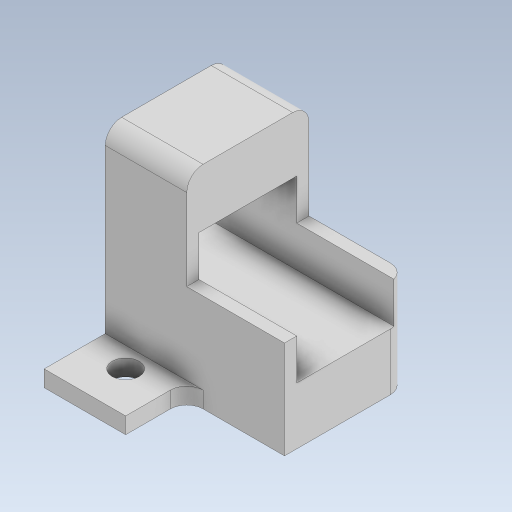
# Autodesk Inventor part: Bracket Motor Pendorong
Saved by Autodesk Inventor 2023.5 (Build 275446000, 446)
## iProperties
Created: 2025-10-12
Part Number: Bracket Motor Pendorong
Material: Generic
Document SubType Name: Modeling
Designer: Guntur
Density: 1 g/cm^3
Appearance: Default
Author: Guntur
Autodesk Inventor part; units mm, degrees
ref_plane "YZ Plane" through (0, 0, 0) normal (1, 0, 0) x (0, 1, 0)
ref_plane "XZ Plane" through (0, 0, 0) normal (0, 1, 0) x (-1, 0, 0)
ref_plane "XY Plane" through (0, 0, 0) normal (0, 0, 1) x (1, 0, 0)
sketch "Sketch1" plane through (0, 0, 0) normal (0, 1, 0) x (-1, 0, 0)
  circle A0 centre (0, -10) radius 1.65
  circle A1 centre (0, 10) radius 1.65
  line L0 (0, 0) -> (-5, 0)
  line L1 (-5, 0) -> (-5, -15)
  line L2 (-5, -15) -> (0, -15)
  line L3 (0, -15) -> (0, 0)
  line L4 (0, 0) -> (5, 0)
  line L5 (5, 0) -> (5, -15)
  line L6 (5, -15) -> (0, -15)
  line L7 (0, -15) -> (0, 0)
  line L8 (5, 0) -> (-5, 0)
  line L9 (-5, 0) -> (-5, 15)
  line L10 (-5, 15) -> (5, 15)
  line L11 (5, 15) -> (5, 0)
  line L12 (5, 7.5) -> (-5, 7.5)
  line L13 (-5, 7.5) -> (-5, -7.5)
  line L14 (-5, -7.5) -> (5, -7.5)
  line L15 (5, -7.5) -> (5, 7.5)
  line L16 (5, 7.5) -> (-5, -7.5) construction
  line L17 (-5, 7.5) -> (5, -7.5) construction
  dimension "d3" = 3.3
  dimension "d6" = 3.3
  constraints: 36 end point, 8 parallel, 4 horizontal, 4 perpendicular, 3 midpoint, 2 centre point, 1 coincident, 1 point on line
  measures "d3" diameter of A0
  measures "d6" diameter of A1
extrude "Extrusion1" add sketch "Sketch1" along normal blind 2 contours A0 L3 L14 L5 L6 | A0 L3 L2 L1 L14 | L9 L10 L11 L12
extrude "Extrusion2" add sketch "Sketch1" along normal blind 24 contours L14 L1 L0 L3 | L3 L4 L5 L14 | L0 L9 L12 L11 L4
sketch "Sketch2" plane through (5, 0, 15) normal (1, 0, 0) x (0, 0, -1)
  line L0 (9, 17) -> (21, 17)
  line L1 (21, 17) -> (21, 7)
  line L2 (21, 7) -> (9, 7)
  line L3 (9, 7) -> (9, 17)
  line L4 (9, 17) -> (21, 7) construction
  line L5 (21, 17) -> (9, 7) construction
  line L6 (7.5, 24) -> (22.5, 24) projected
  line L7 (7.5, 2) -> (7.5, 24) projected
  line L8 (30, 0) -> (0, 0) projected
  line L9 (7.5, 12) -> (22.5, 12)
  line L10 (22.5, 12) -> (22.5, 0)
  line L11 (22.5, 0) -> (7.5, 0)
  line L12 (7.5, 0) -> (7.5, 12)
  point P0 (15, 0)
  point P1 (15, 12)
  point P2 (7.5, 0)
  point P3 (21, 12)
  point P4 (9, 12)
  point P5 (9, 12)
  point P6 (21, 12)
  dimension "d13" = 7
  dimension "d14" = 10
  constraints: 20 end point, 4 parallel, 2 horizontal, 2 midpoint, 2 perpendicular, 2 point on line
  measures "d13" distance between parallel lines of L0 L6
  measures "d14" distance of L0.end L1.end
extrude "Extrusion3" cut sketch "Sketch2" against normal blind 24 contours L0 L1 L9 L3 | L9 L1 L2 L3
extrude "Extrusion4" add sketch "Sketch2" along normal blind 12 contours L3 L2 L1 L9 L10 L8 L12 L7
fillet "Fillet1" radius 2 5 edges at (5, 1, 7.5) (17, 6, -7.5) (5, 1, -7.5) (0, 24, -7.5) (0, 24, 7.5)
body "Solid1"
